KindleStand (Autodesk Fusion 360 design; units mm, degrees)
Autodesk Fusion 360 part; units mm, degrees
sketch "Sketch1" plane through (0, 0, 0) normal (1, 0, 0) x (0, 1, 0)
  line L0 (0, 0) -> (9.7495, 79.4037)
  line L1 (9.7495, 79.4037) -> (18.6825, 78.3069)
  line L2 (18.6825, 78.3069) -> (8.9329, -1.0968)
  line L3 (8.9329, -1.0968) -> (0, 0)
  line L4 (1.5446, -0.1007) -> (5.0446, -0.1007)
  line L5 (5.0446, -0.1007) -> (5.0446, -2.1007)
  line L6 (5.0446, -2.1007) -> (1.5446, -2.1007)
  line L7 (1.5446, -2.1007) -> (1.5446, -0.1007)
  line L8 (0, 140) -> (0, -50)
  line L9 (25, 0) -> (33.3623, 79.5618)
  line L10 (33.3623, 79.5618) -> (43.3075, 78.5165)
  line L11 (43.3075, 78.5165) -> (34.9452, -1.0453)
  line L12 (34.9452, -1.0453) -> (25, 0)
  line L13 (-90, 0) -> (150, 0)
  line L14 (28.2277, -2.2181) -> (31.7277, -2.2181)
  line L15 (31.7277, -2.2181) -> (31.7277, -0.2181)
  line L16 (31.7277, -0.2181) -> (28.2277, -0.2181)
  line L17 (28.2277, -0.2181) -> (28.2277, -2.2181)
  dimension "d1" = 80
  dimension "d2" = 9
  dimension "d9" = 3.5
  dimension "d10" = 2
  dimension "d12" = 80
  dimension "d13" = 10
  dimension "d15" = 97
  dimension "d16" = 96
  dimension "d17" = 25
  dimension "d18" = 3.5
  dimension "d19" = 2
  constraint perpendicular L0 L1
  constraint parallel L0 L2
  constraint parallel L1 L3
  constraint coincident L0.start L3.end
  constraint horizontal L4
  constraint vertical L5
  constraint horizontal L6
  constraint vertical L7
  constraint vertical L8
  constraint perpendicular L9 L10
  constraint parallel L9 L11
  constraint parallel L10 L12
  constraint horizontal L13
  constraint coincident L0.start L8
  constraint coincident L0.start L13
  constraint coincident L9.start L13
  constraint horizontal L14
  constraint vertical L15
  constraint horizontal L16
  constraint vertical L17
  measures "d1" distance of L0.start L0.end
  measures "d2" distance of L0.start L2.end
  measures "d9" distance of L4.start L4.end
  measures "d10" distance of L4.start L6.end
  measures "d12" distance of L9.start L9.end
  measures "d13" distance of L9.start L11.end
  measures "d15" angle of L0 L13
  measures "d16" angle of L9 L13
  measures "d17" distance of L0.start L9.start
  measures "d18" distance of L14.start L14.end
  measures "d19" distance of L14.start L16.end
sketch "Sketch2" plane through (0, 0, 0) normal (1, 0, 0) x (0, 1, 0)
  line L0 (-5.92, 11.2031) -> (64.08, 11.2031)
  line L1 (64.08, 11.2031) -> (64.08, -8.7969)
  line L2 (64.08, -8.7969) -> (-5.92, -8.7969)
  line L3 (-5.92, -8.7969) -> (-5.92, 11.2031)
  dimension "d3" = 70
  dimension "d4" = 20
  constraint horizontal L0
  constraint vertical L1
  constraint horizontal L2
  constraint vertical L3
  measures "d3" distance of L0.start L0.end
  measures "d4" distance of L0.start L2.end
extrude "Extrude1" add sketch "Sketch2" along normal blind 50
extrude "Extrude2" cut sketch "Sketch1" along normal blind 50
fillet "Fillet1" radius 1 4 edges at (25, 5.0446, -0.6194) (25, 1.5446, -0.1897) (25, 31.7277, -0.7071) (25, 28.2277, -0.3392)
fillet "Fillet2" radius 1 4 edges at (25, 10.4432, 11.2031) (25, 36.2326, 11.2031) (25, 26.1775, 11.2031) (25, 1.3756, 11.2031)
fillet "Fillet3" radius 2 1 edges at (25, -5.92, 11.2031)
fillet "Fillet4" radius 17 1 edges at (25, 64.08, 11.2031)
